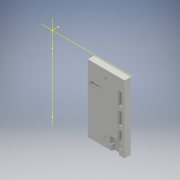
# Autodesk Inventor part: 123
Saved by Autodesk Inventor 2018 (Build 220112000, 112)
## iProperties
Created: 2018-01-17
Part Number: 123
Material: 일반
Document SubType Name: 모델링
Designer: NULL
Density: 1 g/cm^3
Appearance: 기본값
Author: NULL
## iProperties of the stored document 123_3D 인쇄.ipt
Created: 2018-01-20
Part Number: 123_3D 인쇄
Material: 일반
Document SubType Name: Modeling
Designer: NULL
Density: 1 g/cm^3
Appearance: 기본값
Author: NULL
Autodesk Inventor part; units mm, degrees
ref_plane "작업 평면1" through (0, 10, 0) normal (0, 1, 0) x (1, 0, 0)
sketch "스케치3" plane through (0, 10, 0) normal (0, 1, 0) x (1, 0, 0)
  line L0 (113.0685, 80.2704) -> (78.3685, 80.2704)
  line L1 (76.5185, 71.6407) -> (76.5185, 39.8907)
  line L2 (76.5185, 71.6407) -> (62.8185, 71.6407)
  line L3 (78.3685, 80.2704) -> (78.3685, 58.4704)
  line L4 (113.0685, 58.4704) -> (113.0685, 80.2704)
  line L5 (113.0685, 58.4704) -> (78.3685, 58.4704)
  line L6 (108.4435, 113.2704) -> (97.4435, 113.2704)
  line L7 (97.4435, 113.2704) -> (97.4435, 121.7204)
  line L8 (97.4435, 121.7204) -> (108.4435, 121.7204)
  line L9 (108.4435, 121.7204) -> (108.4435, 113.2704)
  line L10 (113.0685, 52.4704) -> (78.3685, 52.4704)
  line L11 (113.0685, 30.6704) -> (113.0685, 52.4704)
  line L12 (62.8185, 39.8907) -> (76.5185, 39.8907)
  line L13 (62.8185, 71.6407) -> (62.8185, 39.8907)
  line L14 (78.3685, 52.4704) -> (78.3685, 30.9204)
  line L15 (113.0685, 30.6704) -> (78.3685, 30.9204)
  line L16 (117.9435, 121.7204) -> (57.9435, 121.7204)
  line L17 (57.9435, 121.7204) -> (57.9435, 11.7204)
  line L18 (117.9435, 11.7204) -> (117.9435, 121.7204)
  line L19 (57.9435, 11.7204) -> (117.9435, 11.7204)
  circle A0 centre (87.9435, 108.2204) radius 2.25
  circle A1 centre (87.9435, 25.2204) radius 2.25
  line L20 (113.0685, 99.0204) -> (108.0685, 99.0204)
  line L21 (108.0685, 90.0204) -> (113.0685, 90.0204)
  line L22 (113.0685, 99.0204) -> (113.0685, 90.0204)
  line L23 (108.0685, 99.0204) -> (108.0685, 90.0204)
  line L24 (71.9185, 39.8907) -> (67.4185, 39.8907)
  line L25 (113.0685, 39.3204) -> (108.0685, 39.3204)
  line L26 (108.0685, 43.8204) -> (113.0685, 43.8204)
  line L27 (71.9185, 44.8907) -> (71.9185, 39.8907)
  line L28 (108.0685, 43.8204) -> (108.0685, 39.3204)
  line L29 (113.0685, 43.8204) -> (113.0685, 39.3204)
  line L30 (71.9185, 44.8907) -> (67.4185, 44.8907)
  line L31 (67.4185, 44.8907) -> (67.4185, 39.8907)
  line L32 (113.0685, 71.6204) -> (113.0685, 67.1204)
  line L33 (113.0685, 86.2704) -> (89.4185, 86.2704)
  line L34 (89.4185, 86.2704) -> (89.4185, 102.7704)
  line L35 (89.4185, 102.7704) -> (113.0685, 102.7704)
  line L36 (113.0685, 102.7704) -> (113.0685, 86.2704)
  line L37 (108.0685, 67.1204) -> (113.0685, 67.1204)
  line L38 (113.0685, 67.1204) -> (113.0685, 71.6204)
  line L39 (113.0685, 71.6204) -> (108.0685, 71.6204)
  line L40 (108.0685, 71.6204) -> (108.0685, 67.1204)
  line L41 (113.0685, 30.6704) -> (108.0685, 30.6704)
  line L42 (108.0685, 30.6704) -> (108.0685, 52.4704)
  line L43 (108.0685, 52.4704) -> (113.0685, 52.4704)
  line L44 (113.0685, 52.4704) -> (113.0685, 30.6704)
  line L45 (113.0685, 58.4704) -> (108.0685, 58.4704)
  line L46 (108.0685, 58.4704) -> (108.0685, 80.2704)
  line L47 (108.0685, 80.2704) -> (113.0685, 80.2704)
  line L48 (113.0685, 80.2704) -> (113.0685, 58.4704)
  line L49 (113.0685, 86.2704) -> (108.0685, 86.2704)
  line L50 (108.0685, 86.2704) -> (108.0685, 102.7704)
  line L51 (108.0685, 102.7704) -> (113.0685, 102.7704)
  line L52 (113.0685, 102.7704) -> (113.0685, 86.2704)
  line L53 (76.5185, 39.8907) -> (62.8185, 39.8907)
  line L54 (62.8185, 39.8907) -> (62.8185, 44.8907)
  line L55 (62.8185, 44.8907) -> (76.5185, 44.8907)
  line L56 (76.5185, 44.8907) -> (76.5185, 39.8907)
  point P0 (0, 0)
  dimension "d8" = 9.5
  constraints: 114 end point, 14 point on line, 12 parallel, 6 horizontal, 6 perpendicular, 2 centre point
  measures "d8" distance of L16.start L8.end
extrude "돌출2" add sketch "스케치3" against normal blind 10 contours L4 L39 L46 L0 | L46 L40 L5 L3 L0 | L4 L37 L40 L39 | L4 L5 L46 L37 | L1 L55 L30 L13 L2 | L1 L12 L27 L55 | L27 L12 L31 L30 | L55 L31 L12 L13 | L9 L16 L18 L19 L17 L7 L6 | L6 L7 L8 L9 | L11 L26 L42 L10 | L42 L28 L15 L14 L10 | L11 L25 L28 L26 | L11 L15 L42 L25 | L41 L42 L15 | A0 | A1 | L22 L21 L23 L20 | L20 L50 L35 L36 | L23 L50 L33 L34 L35 | L36 L33 L50 L21
sketch "스케치4" plane through (0, 10, 0) normal (0, 1, 0) x (1, 0, 0)
  point P0 (0, 0)
extrude "돌출3" cut sketch "스케치3" against normal blind 1.7 contours L4 L39 L46 L0 | L46 L40 L5 L3 L0 | L4 L5 L46 L37 | L1 L55 L30 L13 L2 | L1 L12 L27 L55 | L55 L31 L12 L13 | L11 L26 L42 L10 | L42 L28 L15 L14 L10 | L11 L15 L42 L25 | L20 L50 L35 L36 | L23 L50 L33 L34 L35 | L36 L33 L50 L21
extrude "돌출4" cut sketch "스케치3" against normal through all contours L4 L37 L40 L39 | L27 L12 L31 L30 | L11 L25 L28 L26 | A0 | A1 | L22 L21 L23 L20
sketch "스케치5" plane through (117.9435, 10, -121.7204) normal (0, 0, -1) x (-1, 0, 0)
  point P0 (117.9435, -10)
extrude "돌출5" cut sketch "스케치3" against normal through all contours L6 L7 L8 L9
sketch "스케치6" plane through (0, 0, 0) normal (0, -1, 0) x (1, 0, 0)
  line L0 (57.9435, -121.7204) -> (97.4435, -121.7204) projected
  line L1 (97.4435, -121.7204) -> (57.9435, -121.7204) projected
  line L2 (113.0685, -71.6204) -> (108.0685, -71.6204) projected
  line L3 (113.0685, -80.2704) -> (113.0685, -71.6204) projected
  line L4 (78.3685, -80.2704) -> (113.0685, -80.2704) projected
  line L5 (78.3685, -58.4704) -> (78.3685, -80.2704) projected
  line L6 (113.0685, -58.4704) -> (78.3685, -58.4704) projected
  line L7 (113.0685, -67.1204) -> (113.0685, -58.4704) projected
  line L8 (108.0685, -67.1204) -> (113.0685, -67.1204) projected
  line L9 (108.0685, -71.6204) -> (108.0685, -67.1204) projected
  line L10 (117.9435, -121.7204) -> (108.4435, -121.7204) projected
  line L11 (111.4435, -108.7204) -> (94.443, -108.7204)
  line L12 (111.4435, -108.7204) -> (111.4435, -113.2704)
  line L13 (94.443, -108.7204) -> (94.443, -113.2704)
  line L14 (111.4435, -113.2704) -> (94.443, -113.2704)
  point P0 (0, 0)
  constraints: 8 end point, 2 vertical, 1 perpendicular
sketch "스케치7" plane through (0, 0, 0) normal (0, -1, 0) x (1, 0, 0)
  point P0 (0, 0)
sketch "스케치8" plane through (0, 0, 0) normal (0, -1, 0) x (1, 0, 0)
  point P0 (0, 0)
extrude "돌출6" cut sketch "스케치6" against normal blind 4 contours L12 L14 L13 L11
extrude "돌출7" add sketch "스케치3" against normal blind 6 contours L6 L7 L8 L9
sketch "스케치9" plane through (0, 0, 0) normal (0, -1, 0) x (1, 0, 0)
  line L0 (111.4435, -108.7204) -> (111.4435, -113.2704) projected
  line L1 (111.4435, -108.7204) -> (111.4435, -101.7204)
  line L2 (111.4435, -101.7204) -> (94.443, -101.7204)
  line L3 (94.443, -113.2704) -> (94.443, -108.7204) projected
  line L4 (94.443, -101.7204) -> (94.443, -108.7204)
  line L5 (94.443, -108.7204) -> (111.4435, -108.7204) projected
  line L6 (111.4435, -108.7204) -> (94.443, -108.7204)
  point P0 (0, 0)
  dimension "d25" = 7
  constraints: 8 end point, 2 perpendicular, 1 collinear, 1 vertical
  measures "d25" distance of L0.start L1.end
extrude "돌출8" cut sketch "스케치9" against normal blind 4
sketch "스케치10" plane through (0, 10, 0) normal (0, 1, 0) x (1, 0, 0)
  circle A0 centre (87.9435, 25.2204) radius 2.25 projected
  circle A1 centre (87.9435, 25.2204) radius 3.85
  circle A2 centre (87.9435, 108.2204) radius 2.25 projected
  circle A3 centre (87.9435, 108.2204) radius 3.85
  point P0 (0, 0)
  dimension "d28" = 7.7
  dimension "d29" = 7.7
  constraints: 2 centre point, 2 coincident
  measures "d28" diameter of A1
  measures "d29" diameter of A3
ref_plane "작업 평면2" through (0, 10, 0) normal (0, 1, 0) x (1, 0, 0)
sketch "스케치12" plane through (0, 10, 0) normal (0, 1, 0) x (1, 0, 0)
  point P0 (0, 0)
ref_plane "작업 평면3" through (57.9435, 10, -25.2204) normal (0, 0, 1) x (1, 0, 0)
sketch "스케치13" plane through (57.9435, 10, -25.2204) normal (0, 0, 1) x (1, 0, 0)
  line L0 (30, 0) -> (30, -4)
  line L1 (30, 0) -> (33.65, 0)
  line L2 (27.75, 0) -> (32.25, 0) projected
  line L3 (33.65, 0) -> (30, -4)
  point P0 (-57.9435, -10)
  dimension "d35" = 4
  dimension "d36" = 3.65
  constraints: 6 end point, 1 collinear, 1 vertical
  measures "d35" distance of L0.start L0.end
  measures "d36" distance of L0.start L1.end
sketch "스케치14" plane through (57.9435, 10, -25.2204) normal (0, 0, 1) x (1, 0, 0)
  point P0 (-57.9435, -10)
revolve "회전2" cut sketch "스케치13" angle 360 about axis through (87.9435, 10, -25.2204) along (0, -1, 0)
ref_plane "작업 평면4" through (57.9435, 10, -66.7204) normal (0, 0, 1) x (1, 0, 0)
mirror "미러1" about plane through (57.9435, 10, -66.7204) normal (0, 0, 1) of "회전2"
sketch "스케치15" plane through (0, 0, 0) normal (0, -1, 0) x (1, 0, 0)
  line L0 (108.6612, -121.7204) -> (97.1612, -121.7204)
  line L1 (97.1612, -121.7204) -> (97.1612, -113.2704)
  line L2 (108.6612, -121.7204) -> (108.6612, -113.2704)
  line L3 (97.1612, -113.2704) -> (108.6612, -113.2704)
  line L4 (97.4435, -113.2704) -> (94.443, -113.2704) projected
  point P0 (0, 0)
  constraints: 8 end point, 2 vertical, 1 collinear, 1 horizontal
extrude "돌출9" cut sketch "스케치15" against normal blind 4
extrude "돌출10" cut sketch "스케치3" against normal through all contours L4 L39 L46 L0 | L4 L5 L46 L37 | L1 L12 L27 L55 | L55 L31 L12 L13 | L11 L26 L42 L10 | L11 L15 L42 L25 | L41 L42 L15 | L20 L50 L35 L36 | L36 L33 L50 L21
equation "\"TransitionRadius\" = BendRadius"
equation "\"BendRadius\" = 0.5"
